skadis_bracket_right (Autodesk Fusion 360 design; units mm, degrees)
part number: 2026-09-05-18-11-34-603
Autodesk Fusion 360 part; units mm, degrees
sketch "Plate" plane through (0, 0, 0) normal (0, 1, 0) x (1, 0, 0)
  line L0 (0, 0) -> (5.4, 0)
  line L1 (5.4, 0) -> (5.4, -60)
  line L2 (5.4, -60) -> (0, -60)
  line L3 (0, -60) -> (0, 0)
  dimension "d97" = 5.4
  dimension "d98" = 60
  constraint coincident L0.start L3.end
  constraint horizontal L0
  constraint horizontal L2
  constraint vertical L1
  constraint vertical L3
  measures "d97" horizontal distance of L0.start L1.end
  measures "d98" vertical distance of L0.start L1.end
extrude "Plate (1)" add sketch "Plate" along normal mid plane 24
sketch "Hook profile" plane through (0, 0, 0) normal (0, 1, 0) x (1, 0, 0)
  line L0 (0, -58) -> (-8.3, -58)
  line L1 (-8.3, -58) -> (-8.3, -41)
  line L2 (-8.3, -41) -> (-5.3, -41)
  line L3 (-5.3, -41) -> (-3.8, -42.5)
  line L4 (-3.8, -42.5) -> (-3.8, -53)
  line L5 (-3.8, -53) -> (0, -53)
  line L6 (0, -53) -> (0, -58)
  dimension "d101" = 58
  dimension "d102" = 8.3
  dimension "d103" = 3.8
  dimension "d104" = 5
  dimension "d105" = 10.5
  dimension "d106" = 1.5
  dimension "d107" = 1.5
  constraint horizontal L0
  constraint horizontal L2
  constraint horizontal L5
  constraint vertical L1
  constraint vertical L4
  constraint vertical L6
  constraint coincident origin L6
  measures "d101" vertical distance of origin L0.start
  measures "d102" horizontal distance of L0.start L0.end
  measures "d103" horizontal distance of L4.end L5.end
  measures "d104" vertical distance of L0.start L5.end
  measures "d105" vertical distance of L3.end L4.end
  measures "d106" horizontal distance of L2.end L3.end
  measures "d107" vertical distance of L2.end L3.end
extrude "Hook profile (1)" add sketch "Hook profile" along normal mid plane 2.4
pattern_linear "Hook rows" count 2 spacing 25.4 along (0, 0, -1) count 3 spacing 0 along (0, 0, 1) of "Hook profile (1)"
sketch "Peg profile" plane through (0, 0, 0) normal (0, 1, 0) x (1, 0, 0)
  line L0 (5.4, -45) -> (11.2, -45)
  line L1 (11.2, -45) -> (11.2, -55.4)
  line L2 (11.2, -55.4) -> (10.6, -56)
  line L3 (10.6, -56) -> (10.2, -56)
  line L4 (10.2, -56) -> (10.2, -49)
  line L5 (10.2, -49) -> (5.4, -49)
  line L6 (5.4, -49) -> (5.4, -45)
  dimension "d114" = 5.4
  dimension "d115" = 45
  dimension "d116" = 11.2
  dimension "d117" = 55.4
  dimension "d118" = 10.6
  dimension "d119" = 56
  dimension "d120" = 10.2
  dimension "d121" = 49
  constraint horizontal L0
  constraint horizontal L3
  constraint horizontal L5
  constraint vertical L1
  constraint vertical L4
  constraint vertical L6
  measures "d114" horizontal distance of origin L0.start
  measures "d115" vertical distance of origin L0.start
  measures "d116" horizontal distance of origin L0.end
  measures "d117" vertical distance of origin L1.end
  measures "d118" horizontal distance of origin L2.end
  measures "d119" vertical distance of origin L2.end
  measures "d120" horizontal distance of origin L3.end
  measures "d121" vertical distance of origin L4.end
extrude "Peg profile (1)" add sketch "Peg profile" along normal mid plane 4.8 from surface at -7.52
pattern_linear "Peg rows" count 2 spacing 40 along (0, 0, -1) count 3 spacing 0 along (0, 0, 1) of "Peg profile (1)"
fillet "Peg bearing fillets" radius 1.5 4 edges at (7.8, -9.92, 9) (7.8, -5.12, 9) (7.8, -9.92, 49) (7.8, -5.12, 49)
equation "bracketWidth = 24.0 mm" comment "bracket width across the upright"
equation "plateThickness = 5.4 mm" comment "board rear face sits on this"
equation "plateHeight = 60.0 mm" comment "plate height"
equation "slotWidth = 3.2 mm" comment "measured upright slot width"
equation "slotPitchVertical = 25.4 mm" comment "1 inch, measured"
equation "faceMetalThickness = 2.0 mm" comment "upright face metal"
equation "hookTabWidth = slotWidth - 0.8 mm" comment "blade width through the slot"
equation "hookThroat = faceMetalThickness + 1.8 mm" comment "gap behind the plate"
equation "hookNeckHeight = 5.0 mm" comment "bears on the slot bottom edge"
equation "hookLipThickness = 4.5 mm" comment "lip behind the upright face"
equation "hookLipDrop = 12.0 mm" comment "engagement below the neck"
equation "hookLipChamfer = 1.5 mm" comment "lead-in past slot burrs"
equation "topHookNeckTop = 58.0 mm" comment "top hook row"
equation "hookRows = 2" comment "hook rows (pattern count)"
equation "boardThickness = 4.6 mm" comment "SKADIS panel thickness"
equation "boardSlotWidth = 5.0 mm" comment "SKADIS slot width"
equation "boardSlotHeight = 15.0 mm" comment "SKADIS slot height"
equation "boardPitch = 40.0 mm" comment "SKADIS grid pitch"
equation "pegWidth = boardSlotWidth - 0.2 mm" comment "peg width in the slot"
equation "pegRootLength = boardThickness + 0.2 mm" comment "root through the board"
equation "pegRootHeight = 4.0 mm" comment "slot top edge bears on this"
equation "pegProngThickness = 1.0 mm" comment "prong in front of board"
equation "pegTotalHeight = boardSlotHeight - 4 mm" comment "prong rise above the root, and the lift needed to release"
equation "pegProngChamfer = 0.6 mm" comment "lead-in on the prong top"
equation "pegBearingFillet = 1.5 mm" comment "round on the root top edges the board bears on"
equation "topPegRootZ = 45.0 mm" comment "top peg root, above the plate foot"
equation "pegRows = 2" comment "pegs per bracket (pattern count)"
equation "pegOffsetY = -7.52 mm" comment "offset onto the board's 40 mm grid"
equation "d97 = plateThickness"
equation "d98 = plateHeight"
equation "d99 = bracketWidth"
equation "d101 = topHookNeckTop"
equation "d102 = hookThroat + hookLipThickness"
equation "d103 = hookThroat"
equation "d104 = hookNeckHeight"
equation "d105 = hookLipDrop - hookLipChamfer"
equation "d106 = hookLipChamfer"
equation "d107 = hookLipChamfer"
equation "d108 = hookTabWidth"
equation "d110 = hookRows"
equation "d112 = -slotPitchVertical"
equation "d114 = plateThickness"
equation "d115 = topPegRootZ"
equation "d116 = plateThickness + pegRootLength + pegProngThickness"
equation "d117 = topPegRootZ + pegTotalHeight - pegProngChamfer"
equation "d118 = plateThickness + pegRootLength + pegProngThickness - pegProngChamfer"
equation "d119 = topPegRootZ + pegTotalHeight"
equation "d120 = plateThickness + pegRootLength"
equation "d121 = topPegRootZ + pegRootHeight"
equation "d122 = pegOffsetY"
equation "d123 = pegWidth"
equation "d125 = pegRows"
equation "d127 = -boardPitch"
equation "d130 = pegBearingFillet"
named bodies: "skadis_bracket_right"
